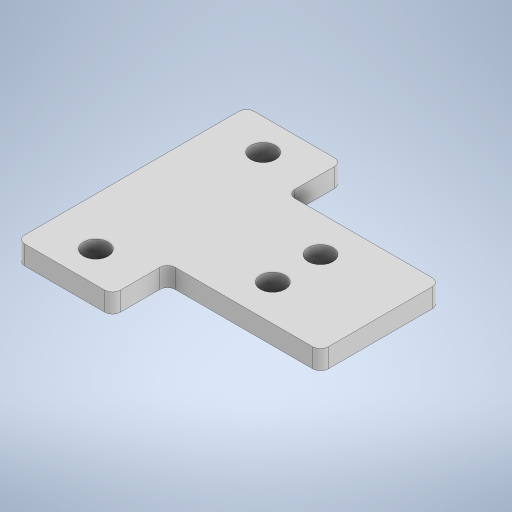
# Autodesk Inventor part: motor_rig_v3
Saved by Autodesk Inventor 2024.2 (Build 282272000, 272)
## iProperties
Created: 2024-02-26
Part Number: motor_rig_v3
Material: Ogólny
Document SubType Name: Modeling
Designer: Konrad
Density: 1 g/cm^3
Appearance: Domyślna
Author: Konrad
Autodesk Inventor part; units mm, degrees
ref_plane "YZ Plane" through (0, 0, 0) normal (1, 0, 0) x (0, 1, 0)
ref_plane "XZ Plane" through (0, 0, 0) normal (0, 1, 0) x (-1, 0, 0)
ref_plane "XY Plane" through (0, 0, 0) normal (0, 0, 1) x (1, 0, 0)
sketch "Szkic1" plane through (0, 0, 0) normal (0, 1, 0) x (-1, 0, 0)
  line L0 (0, 0) -> (52, 0)
  line L1 (52, 0) -> (52, -48)
  line L2 (52, -48) -> (0, -48)
  line L3 (0, -48) -> (0, 0) construction
  line L4 (52, -24) -> (0, -24) construction
  line L5 (32, 0) -> (32, -11.5)
  line L6 (32, -11.5) -> (0, -11.5)
  line L7 (0, -36.5) -> (32, -36.5)
  line L8 (32, -36.5) -> (32, -48)
  line L9 (0, -11.5) -> (0, -36.5)
  circle A0 centre (42, -6.5) radius 2.6
  circle A1 centre (42, -41.5) radius 2.6
  circle A2 centre (17.5, -19) radius 2.6
  circle A3 centre (17.5, -29) radius 2.6
  dimension "d0" = 52
  dimension "d1" = 48
  dimension "d2" = 20
  dimension "d3" = 25
  dimension "d4" = 35
  dimension "d10" = 5.2
  dimension "d11" = 10
  dimension "d12" = 17.5
  dimension "d13" = 10
  constraints: 20 end point, 6 point on line, 4 centre point, 4 perpendicular, 3 equal radius, 2 midpoint, 2 parallel, 2 symmetric about line, 1 collinear, 1 horizontal, 1 other
  measures "d0" distance of L1.end L2.end
  measures "d1" distance of L0.end L1.end
  measures "d2" distance between parallel lines of L1 L5
  measures "d3" distance between parallel lines of L7 L6
  measures "d4" distance of A1.centre A0.centre
  measures "d10" diameter of A2
  measures "d11" distance of A3.centre A2.centre
  measures "d12" distance from line of L9 A2.centre
  measures "d13" distance from line of L5 A0.centre
extrude "Wyciągnięcie proste1" add sketch "Szkic1" along normal blind 4
fillet "Zaokrąglenie1" radius 1.6 8 edges at (-32, 2, -11.5) (0, 2, -11.5) (0, 2, -36.5) (-32, 2, -36.5) (-32, 2, -48) (-52, 2, -48) (-32, 2, 0) (-52, 2, 0)
equation "\"d13\" = 0.5 * d2"
